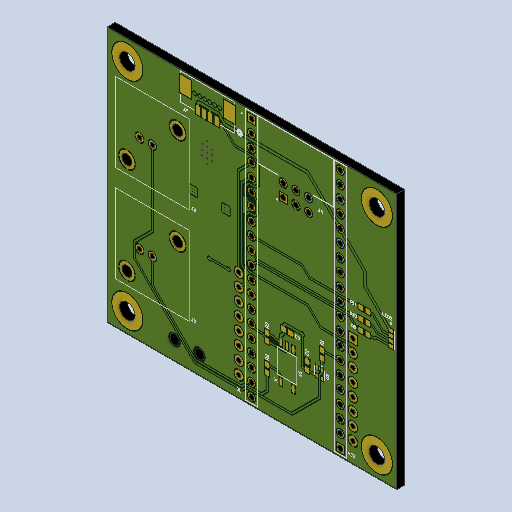
# Autodesk Inventor part: ND_ForagingFeeder_ApplicationBoard_00_BOARD
Saved by Autodesk Inventor 2023.2 (Build 272271000, 271)
## iProperties
Created: 2022-05-04
Part Number: ND_ForagingFeeder_ApplicationBoard_00_BOARD
Material: Generic
Document SubType Name: Modeling
Designer: Graeme
Density: 1 g/cm^3
Appearance: BoardColor
Author: Graeme
Autodesk Inventor part; units mm, degrees
ref_plane "YZ Plane" through (0, 0, 0) normal (1, 0, 0) x (0, 1, 0)
ref_plane "XZ Plane" through (0, 0, 0) normal (0, 1, 0) x (-1, 0, 0)
ref_plane "BoardFrontPlane" through (0, 0, 0) normal (0, 0, 1) x (1, 0, 0)
sketch "Sketch1" plane through (0, 0, 0) normal (0, 0, 1) x (1, 0, 0)
  line L0 (60.5, 48.83) -> (60.5, 100.155)
  line L1 (60.5, 100.155) -> (118.5, 100.155)
  line L2 (118.5, 100.155) -> (118.5, 48.83)
  line L3 (118.5, 48.83) -> (60.5, 48.83)
  constraints: 8 end point
extrude "BoardOutline" add sketch "Sketch1" along normal blind 1.5518
sketch "img_Top" plane through (0, 0, 1.5518) normal (0, 0, 1) x (1, 0, 0)
  line L0 (60.5, 100.155) -> (118.4788, 100.155) construction
  line L1 (118.4788, 100.155) -> (118.4788, 48.83) construction
  line L2 (118.4788, 48.83) -> (60.5, 48.83) construction
  line L3 (60.5, 48.83) -> (60.5, 100.155) construction
  constraints: 2 other
decal "Decal_Top"
sketch "img_Bottom" plane through (0, 0, -1.5518) normal (0, 0, -1) x (1, 0, 0)
  line L0 (60.5, -48.83) -> (118.4788, -48.83) construction
  line L1 (118.4788, -48.83) -> (118.4788, -100.155) construction
  line L2 (118.4788, -100.155) -> (60.5, -100.155) construction
  line L3 (60.5, -100.155) -> (60.5, -48.83) construction
  constraints: 2 other
decal "Decal_Bottom"
sketch "Sketch4" plane through (0, 0, 1.5518) normal (0, 0, 1) x (1, 0, 0)
  point P0 (80.5, 90.33)
hole "U3-26" at (80.5, 90.33, 1.5518) direction (0, 0, -1) diameter 0.25 end through all
sketch "Sketch5" plane through (0, 0, 1.5518) normal (0, 0, 1) x (1, 0, 0)
  point P0 (80.5, 86.33)
hole "U3-16" at (80.5, 86.33, 1.5518) direction (0, 0, -1) diameter 0.25 end through all
sketch "Sketch6" plane through (0, 0, 1.5518) normal (0, 0, 1) x (1, 0, 0)
  point P0 (79.5, 89.33)
hole "U3-23" at (79.5, 89.33, 1.5518) direction (0, 0, -1) diameter 0.25 end through all
sketch "Sketch7" plane through (0, 0, 1.5518) normal (0, 0, 1) x (1, 0, 0)
  point P0 (80.5, 89.33)
hole "U3-24" at (80.5, 89.33, 1.5518) direction (0, 0, -1) diameter 0.25 end through all
sketch "Sketch8" plane through (0, 0, 1.5518) normal (0, 0, 1) x (1, 0, 0)
  point P0 (81.5, 89.33)
hole "U3-25" at (81.5, 89.33, 1.5518) direction (0, 0, -1) diameter 0.25 end through all
sketch "Sketch9" plane through (0, 0, 1.5518) normal (0, 0, 1) x (1, 0, 0)
  point P0 (81.5, 87.33)
hole "U3-19" at (81.5, 87.33, 1.5518) direction (0, 0, -1) diameter 0.25 end through all
sketch "Sketch10" plane through (0, 0, 1.5518) normal (0, 0, 1) x (1, 0, 0)
  point P0 (80.5, 87.33)
hole "U3-18" at (80.5, 87.33, 1.5518) direction (0, 0, -1) diameter 0.25 end through all
sketch "Sketch11" plane through (0, 0, 1.5518) normal (0, 0, 1) x (1, 0, 0)
  point P0 (79.5, 87.33)
hole "U3-17" at (79.5, 87.33, 1.5518) direction (0, 0, -1) diameter 0.25 end through all
sketch "Sketch12" plane through (0, 0, 1.5518) normal (0, 0, 1) x (1, 0, 0)
  point P0 (81.5, 88.33)
hole "U3-22" at (81.5, 88.33, 1.5518) direction (0, 0, -1) diameter 0.25 end through all
sketch "Sketch13" plane through (0, 0, 1.5518) normal (0, 0, 1) x (1, 0, 0)
  point P0 (79.5, 88.33)
hole "U3-20" at (79.5, 88.33, 1.5518) direction (0, 0, -1) diameter 0.25 end through all
sketch "Sketch14" plane through (0, 0, 1.5518) normal (0, 0, 1) x (1, 0, 0)
  point P0 (80.5, 88.33)
hole "U3-21" at (80.5, 88.33, 1.5518) direction (0, 0, -1) diameter 0.25 end through all
sketch "Sketch15" plane through (0, 0, 1.5518) normal (0, 0, 1) x (1, 0, 0)
  point P0 (73.95, 52.5837)
hole "J8-4" at (73.95, 52.5837, 1.5518) direction (0, 0, -1) diameter 1.8542 end through all
sketch "Sketch16" plane through (0, 0, 1.5518) normal (0, 0, 1) x (1, 0, 0)
  point P0 (78.95, 52.5837)
hole "J8-5" at (78.95, 52.5837, 1.5518) direction (0, 0, -1) diameter 1.8542 end through all
sketch "Sketch17" plane through (0, 0, 1.5518) normal (0, 0, 1) x (1, 0, 0)
  point P0 (64.42, 79.075)
hole "J6-SH2" at (64.42, 79.075, 1.5518) direction (0, 0, -1) diameter 2.01 end through all
sketch "Sketch18" plane through (0, 0, 1.5518) normal (0, 0, 1) x (1, 0, 0)
  point P0 (74.58, 89.235)
hole "J6-SH1" at (74.58, 89.235, 1.5518) direction (0, 0, -1) diameter 2.01 end through all
sketch "Sketch19" plane through (0, 0, 1.5518) normal (0, 0, 1) x (1, 0, 0)
  point P0 (66.96, 84.155)
hole "J6-2" at (66.96, 84.155, 1.5518) direction (0, 0, -1) diameter 0.9 end through all
sketch "Sketch20" plane through (0, 0, 1.5518) normal (0, 0, 1) x (1, 0, 0)
  point P0 (69.5, 84.155)
hole "J6-1" at (69.5, 84.155, 1.5518) direction (0, 0, -1) diameter 0.9 end through all
sketch "Sketch21" plane through (0, 0, 1.5518) normal (0, 0, 1) x (1, 0, 0)
  point P0 (69.5, 64.83)
hole "J5-1" at (69.5, 64.83, 1.5518) direction (0, 0, -1) diameter 0.9 end through all
sketch "Sketch22" plane through (0, 0, 1.5518) normal (0, 0, 1) x (1, 0, 0)
  point P0 (66.96, 64.83)
hole "J5-2" at (66.96, 64.83, 1.5518) direction (0, 0, -1) diameter 0.9 end through all
sketch "Sketch23" plane through (0, 0, 1.5518) normal (0, 0, 1) x (1, 0, 0)
  point P0 (74.58, 69.91)
hole "J5-SH1" at (74.58, 69.91, 1.5518) direction (0, 0, -1) diameter 2.01 end through all
sketch "Sketch24" plane through (0, 0, 1.5518) normal (0, 0, 1) x (1, 0, 0)
  point P0 (64.42, 59.75)
hole "J5-SH2" at (64.42, 59.75, 1.5518) direction (0, 0, -1) diameter 2.01 end through all
sketch "Sketch25" plane through (0, 0, 1.5518) normal (0, 0, 1) x (1, 0, 0)
  point P0 (100.815, 90.655)
hole "J4-6" at (100.815, 90.655, 1.5518) direction (0, 0, -1) diameter 1.02 end through all
sketch "Sketch26" plane through (0, 0, 1.5518) normal (0, 0, 1) x (1, 0, 0)
  point P0 (100.815, 88.115)
hole "J4-5" at (100.815, 88.115, 1.5518) direction (0, 0, -1) diameter 1.02 end through all
sketch "Sketch27" plane through (0, 0, 1.5518) normal (0, 0, 1) x (1, 0, 0)
  point P0 (98.275, 90.655)
hole "J4-4" at (98.275, 90.655, 1.5518) direction (0, 0, -1) diameter 1.02 end through all
sketch "Sketch28" plane through (0, 0, 1.5518) normal (0, 0, 1) x (1, 0, 0)
  point P0 (98.275, 88.115)
hole "J4-3" at (98.275, 88.115, 1.5518) direction (0, 0, -1) diameter 1.02 end through all
sketch "Sketch29" plane through (0, 0, 1.5518) normal (0, 0, 1) x (1, 0, 0)
  point P0 (95.735, 90.655)
hole "J4-2" at (95.735, 90.655, 1.5518) direction (0, 0, -1) diameter 1.02 end through all
sketch "Sketch30" plane through (0, 0, 1.5518) normal (0, 0, 1) x (1, 0, 0)
  point P0 (95.735, 88.115)
hole "J4-1" at (95.735, 88.115, 1.5518) direction (0, 0, -1) diameter 1.02 end through all
sketch "Sketch31" plane through (0, 0, 1.5518) normal (0, 0, 1) x (1, 0, 0)
  point P0 (109.695, 52.895)
hole "M1-8" at (109.695, 52.895, 1.5518) direction (0, 0, -1) diameter 0.889 end through all
sketch "Sketch32" plane through (0, 0, 1.5518) normal (0, 0, 1) x (1, 0, 0)
  point P0 (109.695, 55.435)
hole "M1-7" at (109.695, 55.435, 1.5518) direction (0, 0, -1) diameter 0.889 end through all
sketch "Sketch33" plane through (0, 0, 1.5518) normal (0, 0, 1) x (1, 0, 0)
  point P0 (109.695, 57.975)
hole "M1-6" at (109.695, 57.975, 1.5518) direction (0, 0, -1) diameter 0.889 end through all
sketch "Sketch34" plane through (0, 0, 1.5518) normal (0, 0, 1) x (1, 0, 0)
  point P0 (109.695, 60.515)
hole "M1-5" at (109.695, 60.515, 1.5518) direction (0, 0, -1) diameter 0.889 end through all
sketch "Sketch35" plane through (0, 0, 1.5518) normal (0, 0, 1) x (1, 0, 0)
  point P0 (109.695, 63.055)
hole "M1-4" at (109.695, 63.055, 1.5518) direction (0, 0, -1) diameter 0.889 end through all
sketch "Sketch36" plane through (0, 0, 1.5518) normal (0, 0, 1) x (1, 0, 0)
  point P0 (109.695, 65.595)
hole "M1-3" at (109.695, 65.595, 1.5518) direction (0, 0, -1) diameter 0.889 end through all
sketch "Sketch37" plane through (0, 0, 1.5518) normal (0, 0, 1) x (1, 0, 0)
  point P0 (109.695, 68.135)
hole "M1-2" at (109.695, 68.135, 1.5518) direction (0, 0, -1) diameter 0.889 end through all
sketch "Sketch38" plane through (0, 0, 1.5518) normal (0, 0, 1) x (1, 0, 0)
  point P0 (109.695, 70.675)
hole "M1-1" at (109.695, 70.675, 1.5518) direction (0, 0, -1) diameter 0.889 end through all
sketch "Sketch39" plane through (0, 0, 1.5518) normal (0, 0, 1) x (1, 0, 0)
  point P0 (86.835, 52.895)
hole "M1-9" at (86.835, 52.895, 1.5518) direction (0, 0, -1) diameter 0.889 end through all
sketch "Sketch40" plane through (0, 0, 1.5518) normal (0, 0, 1) x (1, 0, 0)
  point P0 (86.835, 55.435)
hole "M1-10" at (86.835, 55.435, 1.5518) direction (0, 0, -1) diameter 0.889 end through all
sketch "Sketch41" plane through (0, 0, 1.5518) normal (0, 0, 1) x (1, 0, 0)
  point P0 (86.835, 57.975)
hole "M1-11" at (86.835, 57.975, 1.5518) direction (0, 0, -1) diameter 0.889 end through all
sketch "Sketch42" plane through (0, 0, 1.5518) normal (0, 0, 1) x (1, 0, 0)
  point P0 (86.835, 60.515)
hole "M1-12" at (86.835, 60.515, 1.5518) direction (0, 0, -1) diameter 0.889 end through all
sketch "Sketch43" plane through (0, 0, 1.5518) normal (0, 0, 1) x (1, 0, 0)
  point P0 (86.835, 63.055)
hole "M1-13" at (86.835, 63.055, 1.5518) direction (0, 0, -1) diameter 0.889 end through all
sketch "Sketch44" plane through (0, 0, 1.5518) normal (0, 0, 1) x (1, 0, 0)
  point P0 (86.835, 65.595)
hole "M1-14" at (86.835, 65.595, 1.5518) direction (0, 0, -1) diameter 0.889 end through all
sketch "Sketch45" plane through (0, 0, 1.5518) normal (0, 0, 1) x (1, 0, 0)
  point P0 (86.835, 68.135)
hole "M1-15" at (86.835, 68.135, 1.5518) direction (0, 0, -1) diameter 0.889 end through all
sketch "Sketch46" plane through (0, 0, 1.5518) normal (0, 0, 1) x (1, 0, 0)
  point P0 (86.835, 70.675)
hole "M1-16" at (86.835, 70.675, 1.5518) direction (0, 0, -1) diameter 0.889 end through all
sketch "Sketch47" plane through (0, 0, 1.5518) normal (0, 0, 1) x (1, 0, 0)
  point P0 (107.155, 50.355)
hole "J2-21" at (107.155, 50.355, 1.5518) direction (0, 0, -1) diameter 1.04 end through all
sketch "Sketch48" plane through (0, 0, 1.5518) normal (0, 0, 1) x (1, 0, 0)
  point P0 (107.155, 52.895)
hole "J2-22" at (107.155, 52.895, 1.5518) direction (0, 0, -1) diameter 1.04 end through all
sketch "Sketch49" plane through (0, 0, 1.5518) normal (0, 0, 1) x (1, 0, 0)
  point P0 (107.155, 55.435)
hole "J2-23" at (107.155, 55.435, 1.5518) direction (0, 0, -1) diameter 1.04 end through all
sketch "Sketch50" plane through (0, 0, 1.5518) normal (0, 0, 1) x (1, 0, 0)
  point P0 (107.155, 57.975)
hole "J2-24" at (107.155, 57.975, 1.5518) direction (0, 0, -1) diameter 1.04 end through all
sketch "Sketch51" plane through (0, 0, 1.5518) normal (0, 0, 1) x (1, 0, 0)
  point P0 (107.155, 60.515)
hole "J2-25" at (107.155, 60.515, 1.5518) direction (0, 0, -1) diameter 1.04 end through all
sketch "Sketch52" plane through (0, 0, 1.5518) normal (0, 0, 1) x (1, 0, 0)
  point P0 (107.155, 63.055)
hole "J2-26" at (107.155, 63.055, 1.5518) direction (0, 0, -1) diameter 1.04 end through all
sketch "Sketch53" plane through (0, 0, 1.5518) normal (0, 0, 1) x (1, 0, 0)
  point P0 (107.155, 65.595)
hole "J2-27" at (107.155, 65.595, 1.5518) direction (0, 0, -1) diameter 1.04 end through all
sketch "Sketch54" plane through (0, 0, 1.5518) normal (0, 0, 1) x (1, 0, 0)
  point P0 (107.155, 68.135)
hole "J2-28" at (107.155, 68.135, 1.5518) direction (0, 0, -1) diameter 1.04 end through all
sketch "Sketch55" plane through (0, 0, 1.5518) normal (0, 0, 1) x (1, 0, 0)
  point P0 (107.155, 70.675)
hole "J2-29" at (107.155, 70.675, 1.5518) direction (0, 0, -1) diameter 1.04 end through all
sketch "Sketch56" plane through (0, 0, 1.5518) normal (0, 0, 1) x (1, 0, 0)
  point P0 (107.155, 73.215)
hole "J2-30" at (107.155, 73.215, 1.5518) direction (0, 0, -1) diameter 1.04 end through all
sketch "Sketch57" plane through (0, 0, 1.5518) normal (0, 0, 1) x (1, 0, 0)
  point P0 (107.155, 75.755)
hole "J2-31" at (107.155, 75.755, 1.5518) direction (0, 0, -1) diameter 1.04 end through all
sketch "Sketch58" plane through (0, 0, 1.5518) normal (0, 0, 1) x (1, 0, 0)
  point P0 (107.155, 78.295)
hole "J2-32" at (107.155, 78.295, 1.5518) direction (0, 0, -1) diameter 1.04 end through all
sketch "Sketch59" plane through (0, 0, 1.5518) normal (0, 0, 1) x (1, 0, 0)
  point P0 (107.155, 80.835)
hole "J2-33" at (107.155, 80.835, 1.5518) direction (0, 0, -1) diameter 1.04 end through all
sketch "Sketch60" plane through (0, 0, 1.5518) normal (0, 0, 1) x (1, 0, 0)
  point P0 (107.155, 83.375)
hole "J2-34" at (107.155, 83.375, 1.5518) direction (0, 0, -1) diameter 1.04 end through all
sketch "Sketch61" plane through (0, 0, 1.5518) normal (0, 0, 1) x (1, 0, 0)
  point P0 (107.155, 85.915)
hole "J2-35" at (107.155, 85.915, 1.5518) direction (0, 0, -1) diameter 1.04 end through all
sketch "Sketch62" plane through (0, 0, 1.5518) normal (0, 0, 1) x (1, 0, 0)
  point P0 (107.155, 88.455)
hole "J2-36" at (107.155, 88.455, 1.5518) direction (0, 0, -1) diameter 1.04 end through all
sketch "Sketch63" plane through (0, 0, 1.5518) normal (0, 0, 1) x (1, 0, 0)
  point P0 (107.155, 90.995)
  dimension "d19" = 0
hole "J2-37" at (107.155, 90.995, 1.5518) direction (0, 0, -1) diameter 1.04 end through all
sketch "Sketch64" plane through (0, 0, 1.5518) normal (0, 0, 1) x (1, 0, 0)
  point P0 (107.155, 93.535)
hole "J2-38" at (107.155, 93.535, 1.5518) direction (0, 0, -1) diameter 1.04 end through all
sketch "Sketch65" plane through (0, 0, 1.5518) normal (0, 0, 1) x (1, 0, 0)
  point P0 (107.155, 96.075)
hole "J2-39" at (107.155, 96.075, 1.5518) direction (0, 0, -1) diameter 1.04 end through all
sketch "Sketch66" plane through (0, 0, 1.5518) normal (0, 0, 1) x (1, 0, 0)
  point P0 (107.155, 98.615)
hole "J2-40" at (107.155, 98.615, 1.5518) direction (0, 0, -1) diameter 1.04 end through all
sketch "Sketch67" plane through (0, 0, 1.5518) normal (0, 0, 1) x (1, 0, 0)
  point P0 (89.375, 98.615)
hole "J1-1" at (89.375, 98.615, 1.5518) direction (0, 0, -1) diameter 1.04 end through all
sketch "Sketch68" plane through (0, 0, 1.5518) normal (0, 0, 1) x (1, 0, 0)
  point P0 (89.375, 96.075)
hole "J1-2" at (89.375, 96.075, 1.5518) direction (0, 0, -1) diameter 1.04 end through all
sketch "Sketch69" plane through (0, 0, 1.5518) normal (0, 0, 1) x (1, 0, 0)
  point P0 (89.375, 93.535)
hole "J1-3" at (89.375, 93.535, 1.5518) direction (0, 0, -1) diameter 1.04 end through all
sketch "Sketch70" plane through (0, 0, 1.5518) normal (0, 0, 1) x (1, 0, 0)
  point P0 (89.375, 90.995)
hole "J1-4" at (89.375, 90.995, 1.5518) direction (0, 0, -1) diameter 1.04 end through all
sketch "Sketch71" plane through (0, 0, 1.5518) normal (0, 0, 1) x (1, 0, 0)
  point P0 (89.375, 88.455)
hole "J1-5" at (89.375, 88.455, 1.5518) direction (0, 0, -1) diameter 1.04 end through all
sketch "Sketch72" plane through (0, 0, 1.5518) normal (0, 0, 1) x (1, 0, 0)
  point P0 (89.375, 85.915)
hole "J1-6" at (89.375, 85.915, 1.5518) direction (0, 0, -1) diameter 1.04 end through all
sketch "Sketch73" plane through (0, 0, 1.5518) normal (0, 0, 1) x (1, 0, 0)
  point P0 (89.375, 83.375)
hole "J1-7" at (89.375, 83.375, 1.5518) direction (0, 0, -1) diameter 1.04 end through all
sketch "Sketch74" plane through (0, 0, 1.5518) normal (0, 0, 1) x (1, 0, 0)
  point P0 (89.375, 80.835)
hole "J1-8" at (89.375, 80.835, 1.5518) direction (0, 0, -1) diameter 1.04 end through all
sketch "Sketch75" plane through (0, 0, 1.5518) normal (0, 0, 1) x (1, 0, 0)
  point P0 (89.375, 78.295)
hole "J1-9" at (89.375, 78.295, 1.5518) direction (0, 0, -1) diameter 1.04 end through all
sketch "Sketch76" plane through (0, 0, 1.5518) normal (0, 0, 1) x (1, 0, 0)
  point P0 (89.375, 75.755)
hole "J1-10" at (89.375, 75.755, 1.5518) direction (0, 0, -1) diameter 1.04 end through all
sketch "Sketch77" plane through (0, 0, 1.5518) normal (0, 0, 1) x (1, 0, 0)
  point P0 (89.375, 73.215)
hole "J1-11" at (89.375, 73.215, 1.5518) direction (0, 0, -1) diameter 1.04 end through all
sketch "Sketch78" plane through (0, 0, 1.5518) normal (0, 0, 1) x (1, 0, 0)
  point P0 (89.375, 70.675)
hole "J1-12" at (89.375, 70.675, 1.5518) direction (0, 0, -1) diameter 1.04 end through all
sketch "Sketch79" plane through (0, 0, 1.5518) normal (0, 0, 1) x (1, 0, 0)
  point P0 (89.375, 68.135)
hole "J1-13" at (89.375, 68.135, 1.5518) direction (0, 0, -1) diameter 1.04 end through all
sketch "Sketch80" plane through (0, 0, 1.5518) normal (0, 0, 1) x (1, 0, 0)
  point P0 (89.375, 65.595)
hole "J1-14" at (89.375, 65.595, 1.5518) direction (0, 0, -1) diameter 1.04 end through all
sketch "Sketch81" plane through (0, 0, 1.5518) normal (0, 0, 1) x (1, 0, 0)
  point P0 (89.375, 63.055)
hole "J1-15" at (89.375, 63.055, 1.5518) direction (0, 0, -1) diameter 1.04 end through all
sketch "Sketch82" plane through (0, 0, 1.5518) normal (0, 0, 1) x (1, 0, 0)
  point P0 (89.375, 60.515)
hole "J1-16" at (89.375, 60.515, 1.5518) direction (0, 0, -1) diameter 1.04 end through all
sketch "Sketch83" plane through (0, 0, 1.5518) normal (0, 0, 1) x (1, 0, 0)
  point P0 (89.375, 57.975)
hole "J1-17" at (89.375, 57.975, 1.5518) direction (0, 0, -1) diameter 1.04 end through all
sketch "Sketch84" plane through (0, 0, 1.5518) normal (0, 0, 1) x (1, 0, 0)
  point P0 (89.375, 55.435)
hole "J1-18" at (89.375, 55.435, 1.5518) direction (0, 0, -1) diameter 1.04 end through all
sketch "Sketch85" plane through (0, 0, 1.5518) normal (0, 0, 1) x (1, 0, 0)
  point P0 (89.375, 52.895)
hole "J1-19" at (89.375, 52.895, 1.5518) direction (0, 0, -1) diameter 1.04 end through all
sketch "Sketch86" plane through (0, 0, 1.5518) normal (0, 0, 1) x (1, 0, 0)
  point P0 (89.375, 50.355)
hole "J1-20" at (89.375, 50.355, 1.5518) direction (0, 0, -1) diameter 1.04 end through all
sketch "Sketch87" plane through (0, 0, 1.5518) normal (0, 0, 1) x (1, 0, 0)
  point P0 (114.5, 52.83)
hole "Free-MH4" at (114.5, 52.83, 1.5518) direction (0, 0, -1) diameter 3.1 end through all
sketch "Sketch88" plane through (0, 0, 1.5518) normal (0, 0, 1) x (1, 0, 0)
  point P0 (114.5, 95.83)
hole "Free-MH3" at (114.5, 95.83, 1.5518) direction (0, 0, -1) diameter 3.1 end through all
sketch "Sketch89" plane through (0, 0, 1.5518) normal (0, 0, 1) x (1, 0, 0)
  point P0 (64.5, 96.155)
hole "Free-MH2" at (64.5, 96.155, 1.5518) direction (0, 0, -1) diameter 3.1 end through all
sketch "Sketch90" plane through (0, 0, 1.5518) normal (0, 0, 1) x (1, 0, 0)
  point P0 (64.5, 52.83)
hole "Free-MH1" at (64.5, 52.83, 1.5518) direction (0, 0, -1) diameter 3.1 end through all
body "Solid1"
